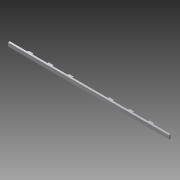
# Autodesk Inventor part: YRail
Saved by Autodesk Inventor 2015 (Build 190159000, 159)
## iProperties
Created: 2016-12-01
Part Number: YRail
Material: Generic
Document SubType Name: Modeling
Designer: Ernest
Density: 1 g/cm^3
Appearance: Default
Author: Ernest
Autodesk Inventor part; units mm, degrees
ref_plane "YZ Plane" through (0, 0, 0) normal (1, 0, 0) x (0, 1, 0)
ref_plane "XZ Plane" through (0, 0, 0) normal (0, 1, 0) x (-1, 0, 0)
ref_plane "XY Plane" through (0, 0, 0) normal (0, 0, 1) x (1, 0, 0)
sketch "Sketch1" plane through (0, 0, 0) normal (0, 0, 1) x (1, 0, 0)
  line L0 (0, 0) -> (1337.4, 0)
  line L1 (1337.4, 0) -> (1337.4, -15)
  line L2 (1337.4, -15) -> (0, -15)
  line L3 (0, -15) -> (0, 0)
  line L4 (167, 59.3402) -> (167, 6.9879) construction
  line L5 (334, 59.3402) -> (334, 6.9879) construction
  line L6 (501, 59.3402) -> (501, 6.9879) construction
  line L7 (1170.4, 15.5437) -> (1170.4, 3.6061) construction
  line L8 (1003.4, 15.5437) -> (1003.4, 3.6061) construction
  line L9 (836.4, 15.5437) -> (836.4, 3.6061) construction
  line L10 (147, 10) -> (187, 10)
  line L11 (187, 10) -> (187, 0)
  line L12 (187, 0) -> (147, 0)
  line L13 (147, 0) -> (147, 10)
  line L14 (314, 10) -> (354, 10)
  line L15 (354, 10) -> (354, 0)
  line L16 (354, 0) -> (314, 0)
  line L17 (314, 0) -> (314, 10)
  line L18 (481, 10) -> (521, 10)
  line L19 (521, 10) -> (521, 0)
  line L20 (521, 0) -> (481, 0)
  line L21 (481, 0) -> (481, 10)
  line L22 (1150.4, 10) -> (1190.4, 10)
  line L23 (1190.4, 10) -> (1190.4, 0)
  line L24 (1190.4, 0) -> (1150.4, 0)
  line L25 (1150.4, 0) -> (1150.4, 10)
  line L26 (983.4, 10) -> (1023.4, 10)
  line L27 (1023.4, 10) -> (1023.4, 0)
  line L28 (1023.4, 0) -> (983.4, 0)
  line L29 (983.4, 0) -> (983.4, 10)
  line L30 (816.4, 10) -> (856.4, 10)
  line L31 (856.4, 10) -> (856.4, 0)
  line L32 (856.4, 0) -> (816.4, 0)
  line L33 (816.4, 0) -> (816.4, 10)
  point P0 (1003.4, 15.5437)
  point P1 (836.4, 15.5437)
  dimension "d0" = 1337.4
  dimension "d1" = 15
  dimension "d2" = 167
  dimension "d5" = 167
  dimension "d10" = 167
  dimension "d13" = 167
  dimension "d18" = 10
  dimension "d19" = 40
  dimension "d20" = 20
  dimension "d23" = 167
  dimension "d28" = 10
  dimension "d29" = 40
  dimension "d30" = 20
  dimension "d33" = 167
  constraints: 68 end point, 7 horizontal, 6 parallel, 4 perpendicular, 2 point on line, 1 vertical, 46 other
  measures "d0" distance of L1.end L2.end
  measures "d1" distance of L0.end L1.end
  measures "d2" distance between parallel lines of L3 L4
  measures "d5" distance of L4.start L5.start
  measures "d10" distance between parallel lines of L1 L7
  measures "d13" distance of L7.start L8.start
  measures "d18" distance between parallel lines of L0 L10
  measures "d19" distance between parallel lines of L11 L13
  measures "d20" distance between parallel lines of L11 L4
  measures "d23" distance of L11.end L15.end
  measures "d28" distance of L22.end L23.end
  measures "d29" distance of L22.start L22.end
  measures "d30" distance between parallel lines of L25 L7
  measures "d33" distance of L7.start point (1003.4, 15.544)
extrude "Extrusion1" add sketch "Sketch1" along normal blind 30
body "Solid1"
